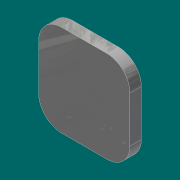
# Autodesk Inventor part: A1-18002-200-02 Foot plate
Saved by Autodesk Inventor 2017 (Build 210142000, 142)
## iProperties
Created: 2018-01-24
Part Number: A1-18002-200-02 Foot plate
Material: Steel, Mild
Document SubType Name: Modeling
Designer: Graeme_Van_Dongen
Density: 7.85 g/cm^3
Appearance: Steel
Mass: 122.228 g
Surface Area: 60.5842 cm^2
Volume: 15.5705 cm^3
Description: 2" x 2" x 1/4" PLATE, 44W
Author: Graeme_Van_Dongen
Autodesk Inventor part; units mm, degrees
ref_plane "YZ Plane" through (0, 0, 0) normal (1, 0, 0) x (0, 1, 0)
ref_plane "XZ Plane" through (0, 0, 0) normal (0, 1, 0) x (-1, 0, 0)
ref_plane "XY Plane" through (0, 0, 0) normal (0, 0, 1) x (1, 0, 0)
sketch "Sketch1" plane through (0, 0, 0) normal (0, 0, 1) x (1, 0, 0)
  line L0 (-12.7, -25.497) -> (12.7, -25.497)
  line L1 (25.4, -12.797) -> (25.4, 12.797)
  line L2 (12.7, 25.497) -> (-12.7, 25.497)
  line L3 (-25.4, 12.797) -> (-25.4, -12.797)
  line L4 (-25.4, -25.497) -> (25.4, 25.497) construction
  line L5 (25.4, -25.497) -> (-25.4, 25.497) construction
  arc A0 (-12.7, 25.497) -> (-25.4, 12.797) centre (-12.7, 12.797) ccw
  arc A1 (25.4, 12.797) -> (12.7, 25.497) centre (12.7, 12.797) ccw
  arc A2 (12.7, -25.497) -> (25.4, -12.797) centre (12.7, -12.797) ccw
  arc A3 (-25.4, -12.797) -> (-12.7, -25.497) centre (-12.7, -12.797) ccw
  point P0 (0, 0)
  dimension "d0" = 50.8
  dimension "d1" = 50.9941
  dimension "d2" = 12.7
  constraints: 12 end point, 8 point on circle, 8 point on line, 8 tangent, 4 centre point, 3 equal radius, 2 midpoint, 2 parallel, 1 horizontal, 1 perpendicular
  measures "d0" distance of L5.end L4.end
  measures "d1" distance of L5.start L4.end
  measures "d2" radius of A0
extrude "Extrusion1" add sketch "Sketch1" along normal blind 6.35
equation "\"d1\" = 1.00382 * d0"
body "Solid1"
